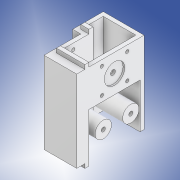
# Autodesk Inventor part: BA003
Saved by Autodesk Inventor 2017 (Build 210142000, 142)
## iProperties
Created: 2017-06-15
Part Number: BA003
Material: ABS Plastic
Document SubType Name: Modeling
Designer: zallen
Density: 1.06 g/cm^3
Appearance: CR White
Author: zallen
Autodesk Inventor part; units mm, degrees
ref_plane "YZ Plane" through (0, 0, 0) normal (1, 0, 0) x (0, 1, 0)
ref_plane "XZ Plane" through (0, 0, 0) normal (0, 1, 0) x (-1, 0, 0)
ref_plane "XY Plane" through (0, 0, 0) normal (0, 0, 1) x (1, 0, 0)
sketch "Sketch1" plane through (0, 0, 0) normal (0, 0, 1) x (1, 0, 0)
  line L0 (0, 0) -> (40, 0)
  line L1 (40, 0) -> (40, 100)
  line L2 (40, 100) -> (0, 100)
  line L3 (0, 100) -> (0, 0)
  dimension "d0" = 40
  dimension "d1" = 100
  constraints: 8 end point, 2 parallel, 1 horizontal, 1 perpendicular
  measures "d0" distance of L2.end L1.end
  measures "d1" distance of L1.end L0.end
extrude "Extrusion1" add sketch "Sketch1" along normal blind 45
sketch "Sketch2" plane through (0, 0, 0) normal (0, 0, -1) x (-1, 0, 0)
  line L0 (-40, 0) -> (-40, 100) projected
  line L1 (-40, 100) -> (10, 100)
  line L2 (10, 100) -> (10, 0)
  line L3 (10, 0) -> (-40, 0)
  line L4 (-40, 0) -> (-40, 100)
  point P0 (0, 0)
  dimension "d4" = 10
  constraints: 8 end point, 2 parallel, 1 horizontal, 1 horizontal alignment, 1 perpendicular
  measures "d4" distance from line of point (0, 0) L2
extrude "Extrusion2" add sketch "Sketch2" along normal blind 37.5
sketch "Sketch3" plane through (40, 0, 45) normal (1, 0, 0) x (0, 0, -1)
  line L0 (82.5, 100) -> (0, 100) projected
  line L1 (0, 0) -> (0, 100) projected
  line L2 (82.5, 0) -> (0, 0) projected
  line L3 (82.5, 100) -> (82.5, 0) projected
  line L4 (5, 5) -> (5, 95)
  line L5 (5, 95) -> (77.5, 95)
  line L6 (77.5, 95) -> (77.5, 5)
  line L7 (77.5, 5) -> (5, 5)
  point P0 (45, 0)
  dimension "d7" = 5
  constraints: 8 end point, 3 other
  measures "d7" distance between parallel lines of L2 L7
extrude "Extrusion3" cut sketch "Sketch3" against normal blind 35 contours L4 L5 L6 L7
sketch "Sketch4" plane through (5, 0, 45) normal (1, 0, 0) x (0, 0, -1)
  line L0 (45, 100) -> (45, 0) projected
  line L1 (45, 100) -> (82.5, 100) projected
  line L2 (82.5, 0) -> (82.5, 100) projected
  line L3 (45, 0) -> (82.5, 0) projected
  line L4 (50, 5) -> (50, 95)
  line L5 (50, 95) -> (77.5, 95)
  line L6 (77.5, 95) -> (77.5, 5)
  line L7 (77.5, 5) -> (50, 5)
  point P0 (45, 0)
  dimension "d10" = 5
  constraints: 8 end point, 3 other
  measures "d10" distance between parallel lines of L0 L4
extrude "Extrusion4" cut sketch "Sketch4" against normal blind 10 contours L4 L5 L6 L7
sketch "Sketch5" plane through (0, 0, 45) normal (0, -1, 0) x (1, 0, 0)
  line L0 (0, 0) -> (40, 0) projected
  line L1 (0, -45) -> (0, 0) projected
  line L2 (-10, -45) -> (0, -45) projected
  line L3 (-10, -45) -> (-10, -82.5) projected
  line L4 (40, -82.5) -> (-10, -82.5) projected
  line L5 (40, -77.5) -> (-5, -77.5)
  line L6 (-5, -77.5) -> (-5, -50)
  line L7 (-5, -50) -> (5, -50)
  line L8 (5, -50) -> (5, -5)
  line L9 (5, -5) -> (40, -5)
  line L10 (40, -77.5) -> (40, -5)
  line L11 (40, -82.5) -> (40, 0) projected
  dimension "d13" = 5
  constraints: 12 end point, 1 collinear, 4 other
  measures "d13" distance between parallel lines of L4 L5
extrude "Extrusion5" cut sketch "Sketch5" against normal through all contours L10 L5 L6 L7 L8 L9
sketch "Sketch6" plane through (0, 100, 45) normal (0, 1, 0) x (1, 0, 0)
  line L0 (0, 45) -> (0, 0) projected
  line L1 (0, 0) -> (40, 0)
  line L2 (40, 0) -> (40, 10)
  line L3 (40, 10) -> (0, 10)
  line L4 (0, 10) -> (0, 0)
  dimension "d16" = 40
  dimension "d17" = 10
  constraints: 8 end point, 2 parallel, 1 horizontal, 1 perpendicular
  measures "d16" distance of L3.end L2.end
  measures "d17" distance of L2.end L1.end
extrude "Extrusion6" add sketch "Sketch6" against normal blind 100
sketch "Sketch8" plane through (40, 100, 35) normal (0, 0, -1) x (-1, 0, 0)
  line L0 (35, 0) -> (35, -100) projected
  line L1 (0, 0) -> (35, 0) projected
  line L2 (0, 0) -> (0, -100) projected
  line L3 (35, -100) -> (0, -100) projected
  line L4 (35, -105) -> (0, -105)
  line L5 (0, -105) -> (0, 5)
  line L6 (0, 5) -> (35, 5)
  line L7 (35, 5) -> (35, -105)
  point P0 (40, -100)
  dimension "d20" = 5
  dimension "d21" = 5
  constraints: 8 end point, 2 parallel, 1 horizontal, 1 perpendicular, 1 point on line
  measures "d20" distance between parallel lines of L4 L3
  measures "d21" distance between parallel lines of L1 L6
extrude "Extrusion7" add sketch "Sketch8" along normal blind 5
sketch "Sketch10" plane through (5, 0, -5) normal (0, 0, -1) x (-1, 0, 0)
  line L0 (0, 0) -> (0, 100) projected
  line L1 (10, 0) -> (0, 0) projected
  line L2 (10, 0) -> (10, 100) projected
  line L3 (0, 100) -> (10, 100) projected
  line L4 (-35, -5) -> (0, -5) projected
  line L5 (10, 0) -> (0, 0)
  line L6 (0, 0) -> (0, -5)
  line L7 (0, -5) -> (10, -5)
  line L8 (10, -5) -> (10, 0)
  line L9 (0, 105) -> (0, 100) projected
  line L10 (10, 100) -> (0, 100)
  line L11 (0, 100) -> (0, 105)
  line L12 (0, 105) -> (10, 105)
  line L13 (10, 105) -> (10, 100)
  point P0 (5, 0)
  constraints: 16 end point, 4 parallel, 2 horizontal, 2 perpendicular
extrude "Extrusion8" add sketch "Sketch10" along normal blind 5
sketch "Sketch22" plane through (40, 0, -37.5) normal (1, 0, 0) x (0, 0, -1)
  line L0 (-67.5, 105) -> (-67.5, -5) projected
  line L1 (-5, 100) -> (-5, 0) projected
  line L2 (-5, 100) -> (-67.5, 100)
  line L3 (-67.5, 100) -> (-67.5, 55)
  line L4 (-67.5, 55) -> (-5, 55)
  line L5 (-5, 55) -> (-5, 100)
  line L6 (-20.75, 62) -> (-51.75, 62) construction
  line L7 (-51.75, 62) -> (-51.75, 93) construction
  line L8 (-51.75, 93) -> (-20.75, 93) construction
  line L9 (-20.75, 93) -> (-20.75, 62) construction
  circle A0 centre (-51.75, 62) radius 1.5
  circle A1 centre (-51.75, 93) radius 1.5
  circle A2 centre (-20.75, 93) radius 1.5
  circle A3 centre (-20.75, 62) radius 1.5
  circle A4 centre (-36.25, 77.5) radius 3
  point P0 (-37.5, 0)
  point P1 (-51.75, 77.5)
  point P2 (-67.5, 77.5)
  point P3 (-36.25, 62)
  point P4 (-36.25, 55)
  dimension "d70" = 45
  dimension "d71" = 31
  dimension "d72" = 31
  dimension "d73" = 3
  dimension "d74" = 3
  dimension "d75" = 3
  dimension "d76" = 3
  dimension "d77" = 6
  constraints: 16 end point, 5 centre point, 4 coincident, 4 midpoint, 4 parallel, 2 horizontal, 2 horizontal alignment, 2 perpendicular, 2 vertical alignment, 1 point on line
  measures "d70" distance of L3.end L2.end
  measures "d71" distance of L7.end L8.end
  measures "d72" distance of L6.end L7.end
  measures "d73" diameter of A0
  measures "d74" diameter of A1
  measures "d75" diameter of A2
  measures "d76" diameter of A3
  measures "d77" diameter of A4
extrude "Extrusion19" add sketch "Sketch22" against normal blind 5
sketch "Sketch23" plane through (40, 0, 45) normal (1, 0, 0) x (0, 0, -1)
  circle A0 centre (46.25, 77.5) radius 3 projected
  circle A1 centre (46.25, 77.5) radius 12.5
  point P0 (45, 0)
  dimension "d80" = 25
  constraints: 1 centre point, 1 coincident
  measures "d80" diameter of A1
extrude "Extrusion20" cut sketch "Sketch23" against normal blind 2
sketch "Sketch24" plane through (40, 0, 45) normal (1, 0, 0) x (0, 0, -1)
  circle A0 centre (30.75, 62) radius 1.5 projected
  circle A1 centre (30.75, 93) radius 1.5 projected
  circle A2 centre (61.75, 93) radius 1.5 projected
  circle A3 centre (61.75, 62) radius 1.5 projected
  circle A4 centre (30.75, 62) radius 2
  circle A5 centre (30.75, 93) radius 2
  circle A6 centre (61.75, 93) radius 2
  circle A7 centre (61.75, 62) radius 2
  point P0 (45, 0)
  dimension "d83" = 4
  dimension "d84" = 4
  dimension "d85" = 4
  dimension "d86" = 4
  constraints: 4 centre point, 4 coincident
  measures "d83" diameter of A4
  measures "d84" diameter of A5
  measures "d85" diameter of A6
  measures "d86" diameter of A7
extrude "Extrusion21" cut sketch "Sketch24" against normal through all contours A0 | A1 | A2 | A3 | A4 | A5 | A6 | A7
sketch "Sketch25" plane through (5, 0, 45) normal (1, 0, 0) x (0, 0, -1)
  circle A0 centre (32.5, 25) radius 10
  circle A1 centre (32.5, 25) radius 2.5
  line L0 (50, 0) -> (15, 0) projected
  line L1 (15, 55) -> (15, -5) projected
  circle A2 centre (66.25, 25) radius 2.5
  circle A3 centre (66.25, 25) radius 10
  line L2 (77.5, 0) -> (55, 0) projected
  point P0 (32.5, 0)
  point P1 (15, 25)
  point P2 (66.25, 0)
  dimension "d89" = 20
  dimension "d90" = 5
  dimension "d93" = 5
  dimension "d94" = 20
  constraints: 4 centre point, 3 midpoint, 2 coincident, 2 horizontal alignment, 2 vertical alignment
  measures "d89" diameter of A0
  measures "d90" diameter of A1
  measures "d93" diameter of A2
  measures "d94" diameter of A3
extrude "Extrusion22" add sketch "Sketch25" along normal blind 35
sketch "Sketch26" plane through (-5, 0, 45) normal (1, 0, 0) x (0, 0, -1)
  circle A0 centre (66.25, 25) radius 10 projected
  circle A1 centre (66.25, 25) radius 2.5 projected
  point P0 (45, 0)
extrude "Extrusion23" add sketch "Sketch26" along normal blind 10
body "Solid1"
